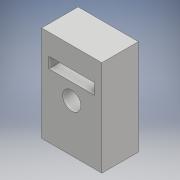
# Autodesk Inventor part: armpart3
Saved by Autodesk Inventor 2018.3 (Build 223284000, 284)
## iProperties
Created: 2019-11-01
Part Number: armpart3
Material: 一般
Document SubType Name: Modeling
Designer: Eiji Nishizawa
Density: 1 g/cm^3
Appearance: 既定
Author: Eiji Nishizawa
Autodesk Inventor part; units mm, degrees
ref_plane "YZ Plane" through (0, 0, 0) normal (1, 0, 0) x (0, 1, 0)
ref_plane "XZ Plane" through (0, 0, 0) normal (0, 1, 0) x (-1, 0, 0)
ref_plane "XY Plane" through (0, 0, 0) normal (0, 0, 1) x (1, 0, 0)
sketch "スケッチ1" plane through (0, 0, 0) normal (0, 1, 0) x (-1, 0, 0)
  line L0 (7.6573, 10.2043) -> (-8.8427, 10.2043)
  line L1 (-8.8427, 10.2043) -> (-8.8427, -15.9957)
  line L2 (-8.8427, -15.9957) -> (7.6573, -15.9957)
  line L3 (7.6573, -15.9957) -> (7.6573, 10.2043)
  line L4 (5.6573, 8.2043) -> (-6.8427, 8.2043)
  line L5 (-6.8427, 8.2043) -> (-6.8427, -13.9957)
  line L6 (-6.8427, -13.9957) -> (5.6573, -13.9957)
  line L7 (5.6573, -13.9957) -> (5.6573, 8.2043)
  line L8 (5.6573, 8.2043) -> (0.5388, 8.2043)
  line L9 (0.5388, -13.9957) -> (5.6573, -13.9957)
  line L10 (5.6573, -13.9957) -> (5.6573, 8.2043)
  circle A0 centre (-0.5927, -2.8957) radius 2.5
  line L11 (-6.8427, 4.5043) -> (5.6573, 4.5043)
  line L12 (5.6573, 4.5043) -> (5.6573, 1.5043)
  line L13 (5.6573, 1.5043) -> (-6.8427, 1.5043)
  line L14 (-6.8427, 1.5043) -> (-6.8427, 4.5043)
  point P0 (0, 0)
  dimension "d0" = 12.5
  dimension "d1" = 22.2
  dimension "d2" = 2
  dimension "d3" = 2
  dimension "d4" = 2
  dimension "d5" = 2
  dimension "d6" = 3.7
  dimension "d7" = 3
  dimension "d8" = 5
  dimension "d9" = 6.25
  dimension "d11" = 13.1
  dimension "d12" = 13.1
  dimension "d17" = 6.25
  constraints: 30 end point, 7 parallel, 4 horizontal, 3 perpendicular, 3 point on line, 1 centre point
  measures "d0" distance of L4.start L4.end
  measures "d1" distance of L6.end L4.start
  measures "d2" distance between parallel lines of L0 L4
  measures "d3" distance between parallel lines of L2 L6
  measures "d4" distance between parallel lines of L3 L7
  measures "d5" distance between parallel lines of L1 L5
  measures "d6" distance between parallel lines of L8 L11
  measures "d7" distance between parallel lines of L11 L13
  measures "d8" diameter of A0
  measures "d9" distance from line of L5 A0.centre
  measures "d11" distance from line of L0 A0.centre
  measures "d12" distance from line of L2 A0.centre
  measures "d17" distance from line of L7 A0.centre
extrude "押し出し1" add sketch "スケッチ1" along normal blind 5 contours L3 L2 L1 L0
extrude "押し出し2" add sketch "スケッチ1" against normal blind 5 contours L3 L2 L1 L0 | L7 L11 L5 L4 | L7 L6 L5 L13
sketch "スケッチ2" plane through (0, 5, 0) normal (0, 1, 0) x (1, 0, 0)
  line L0 (8.8427, -10.2043) -> (8.8427, 15.9957) projected
  line L1 (8.8427, 15.9957) -> (-7.6728, 15.9957)
  line L2 (-7.6728, 15.9957) -> (-7.6728, 14.001)
  line L3 (-7.6728, 14.001) -> (8.8427, 14.001)
  line L4 (8.8427, 14.001) -> (8.8427, 15.9957)
  point P0 (0, 0)
  constraints: 8 end point, 2 parallel, 1 horizontal, 1 perpendicular
